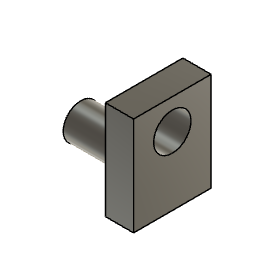
Assembled Crankshaft Model (Autodesk Fusion 360 archive; units mm, degrees)
design "Square Crank Proto"
Autodesk Fusion 360 part; units mm, degrees
box "BoxPrimitive1" add length 14 width 11 height 4 placed x (0, 0, 1) y (0, -1, 0) z (1, 0, 0) at (0, 11, 0) makes body 1
cylinder "CylinderPrimitive1" add diameter 4.8 height 9 placed x (0, 0, -1) y (0, 1, 0) z (1, 0, 0) at (4, 5.5, 13) separate body makes body 2
move_body "Move1" bodies 2 to x (1, 0, 0) y (0, 1, 0) z (0, 0, 1) at (0, 0, -2)
ref_plane "WorkPlane1" through (2, 5.5, 7) normal (0, 1, 0) x (-1, 0, 0)
cylinder "CylinderPrimitive2" add diameter 5 height 2 placed x (0, 0, -1) y (0, 1, 0) z (1, 0, 0) at (4, 5, 2) separate body makes body 3
move_body "Move2" bodies 3 to x (1, 0, 0) y (0, 1, 0) z (0, 0, 1) at (0, 0, 2)
move_body "Move3" bodies 3 to x (1, 0, 0) y (0, 1, 0) z (0, 0, 1) at (0, 0.5, 0)
move_body "Move4" bodies 3 to x (1, 0, 0) y (0, 1, 0) z (0, 0, 1) at (0, 0, 0.5)
move_body "Move5" bodies 2 to x (1, 0, 0) y (0, 1, 0) z (0, 0, 1) at (0, 0, -1.4)
extrude "Extrude1" cut 1 faces at (6, 5.9821, 5.0196) along direction (-1, 0, 0) blind 10 on bodies 3 bodies 1 3
cylinder "CylinderPrimitive3" add diameter 5 height -13 placed x (0, 0, -1) y (0, 1, 0) z (1, 0, 0) at (4, 5.5, 4.5) bodies 1 3
